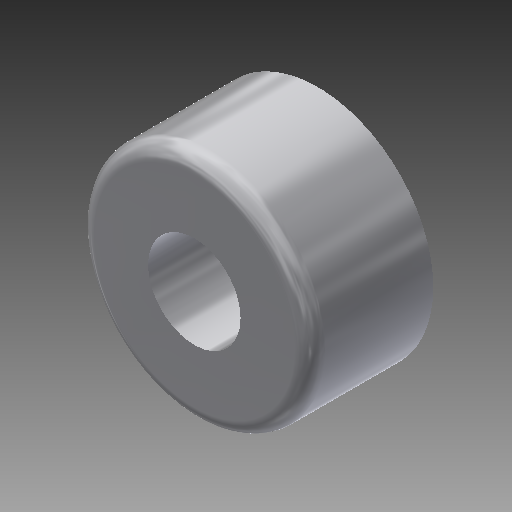
# Autodesk Inventor part: セットカラーΦ6
Saved by Autodesk Inventor 2017.3 (Build 213256000, 256)
## iProperties
Created: 2016-05-05
Part Number: セットカラーΦ6
Material: アセタール樹脂、白
Document SubType Name: Modeling
Designer: 大空
Density: 1.425 g/cm^3
Appearance: 滑らか - 白
Mass: 1.67824 g
Surface Area: 8.03997 cm^2
Volume: 1.17771 cm^3
Author: 大空
Autodesk Inventor part; units mm, degrees
ref_plane "YZ Plane" through (0, 0, 0) normal (1, 0, 0) x (0, 1, 0)
ref_plane "XZ Plane" through (0, 0, 0) normal (0, 1, 0) x (-1, 0, 0)
ref_plane "XY Plane" through (0, 0, 0) normal (0, 0, 1) x (1, 0, 0)
sketch "スケッチ1" plane through (0, 0, 0) normal (0, 0, 1) x (1, 0, 0)
  circle A0 centre (0, 0) radius 3
  circle A1 centre (0, 0) radius 7.5
  dimension "d0" = 6
  dimension "d1" = 15
  constraints: 2 centre point, 2 coincident
  measures "d0" diameter of A0
  measures "d1" diameter of A1
extrude "押し出し1" add sketch "スケッチ1" along normal blind 8
fillet "フィレット1" radius 1 1 edges at (-7.5, 0, 8)
